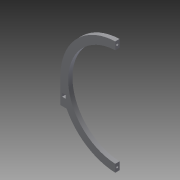
# Autodesk Inventor part: TopfemaleHoopSection_v3
Saved by Autodesk Inventor 2013 (Build 170138000, 138)
## iProperties
Created: 2013-01-17
Part Number: TopfemaleHoopSection_v3
Material: Generic
Document SubType Name: Modeling
Designer: motoennies
Density: 1 g/cm^3
Author: motoennies
Autodesk Inventor part; units mm, degrees
ref_plane "YZ Plane" through (0, 0, 0) normal (1, 0, 0) x (0, 1, 0)
ref_plane "XZ Plane" through (0, 0, 0) normal (0, 1, 0) x (-1, 0, 0)
ref_plane "XY Plane" through (0, 0, 0) normal (0, 0, 1) x (1, 0, 0)
sketch "Sketch1" plane through (0, 0, 0) normal (0, 0, 1) x (1, 0, 0)
  arc A0 (-6.35, 145.9119) -> (0, -146.05) centre (0, 0) ccw
  line L0 (-168.91, 0) -> (168.91, 0) construction
  line L1 (0, -146.05) -> (0, -168.91) construction
  line L2 (-168.91, 0) -> (-168.91, -76.2)
  line L3 (-168.91, -76.2) -> (-150.7453, -76.2)
  line L4 (0, 0) -> (0, -47.2694) construction
  line L5 (0, -47.2694) -> (-158.75, -47.2694) construction
  line L6 (-158.75, -42.5069) -> (-153.67, -42.5069)
  line L7 (-153.67, -42.5069) -> (-153.67, -52.0319)
  line L8 (-153.67, -52.0319) -> (-163.83, -52.0319)
  line L9 (-163.83, -52.0319) -> (-163.83, -42.5069)
  line L10 (-163.83, -42.5069) -> (-158.75, -42.5069)
  arc A1 (-150.7453, -76.2) -> (-6.35, -168.7906) centre (0, 0) ccw
  arc A2 (-6.35, 168.7906) -> (-168.91, 0) centre (0, 0) ccw
  line L11 (-6.35, -145.9119) -> (-6.35, -151.13)
  line L12 (-6.35, -161.29) -> (-6.35, -168.7906)
  line L13 (-6.35, -145.9119) -> (-6.35, -151.13)
  line L14 (-6.35, -161.29) -> (-6.35, -168.7906)
  line L15 (-6.35, 168.7906) -> (-6.35, 161.29)
  line L16 (-6.35, 151.13) -> (-6.35, 145.9119)
  line L17 (-6.35, -168.7906) -> (-6.35, -161.29)
  line L18 (-6.35, -151.13) -> (-6.35, -145.9119)
  line L19 (-6.35, 161.29) -> (-6.35, 151.13)
  line L20 (-6.35, -151.13) -> (-6.35, -161.29)
  point P0 (0, 161.29)
  point P1 (0, -151.13)
  point P2 (0, -161.29)
  dimension "d0" = 292.1
  dimension "d8" = 76.2
  dimension "d9" = 47.2694
  dimension "d10" = 158.75
  dimension "d12" = 4.7625
  dimension "d13" = 5.08
  dimension "d14" = 9.525
  dimension "d15" = 10.16
  dimension "d17" = 5.08
  dimension "d22" = 22.8787
  dimension "d23" = 24.1681
  dimension "d26" = 168.91
  constraints: 42 end point, 7 point on circle, 6 collinear, 6 perpendicular, 4 symmetric about line, 3 centre point, 2 coincident, 1 line through centre, 1 parallel, 1 tangent, 1 vertical, 1 other
  measures "d0" diameter of A0
  measures "d8" distance of L0.start L2.end
  measures "d9" distance of L4.start L4.end
  measures "d10" distance of L4.end L5.end
  measures "d12" distance of L5.end L6.start
  measures "d13" distance of L6.start L6.end
  measures "d14" distance of L6.end L7.end
  measures "d15" distance of L7.end L8.end
  measures "d17" distance between parallel lines of L2 L9
  measures "d22" distance of L11.start L12.end
  measures "d23" distance between parallel lines of L3 L8
  measures "d26" distance from line of point (0, 0) L2
extrude "Extrusion1" add sketch "Sketch1" along normal blind 12.7
sketch "Sketch2" plane through (-6.35, 145.9119, 0) normal (1, 0, 0) x (0, 0, -1)
  line L0 (0, 0) -> (0, 22.8787) projected
  line L1 (0, 22.8787) -> (-12.7, 22.8787) projected
  line L2 (0, 0) -> (-12.7, 0) projected
  circle A0 centre (-6.35, 11.436) radius 3.175
  line L3 (0, -145.9119) -> (96.3473, -145.9119) construction
  line L4 (96.3473, -145.9119) -> (-165.7611, -145.9119) construction
  circle A1 centre (-6.35, -303.2598) radius 3.175
  dimension "d27" = 6.35
  dimension "d28" = 11.4427
  dimension "d29" = 6.35
  constraints: 4 end point, 2 centre point, 1 collinear, 1 parallel, 1 symmetric about line, 1 other
  measures "d27" diameter of A0
  measures "d28" distance from line of L1 A0.centre
  measures "d29" distance from line of L0 A0.centre
extrude "Extrusion2" cut sketch "Sketch2" against normal blind 6.35
body "Solid1"
